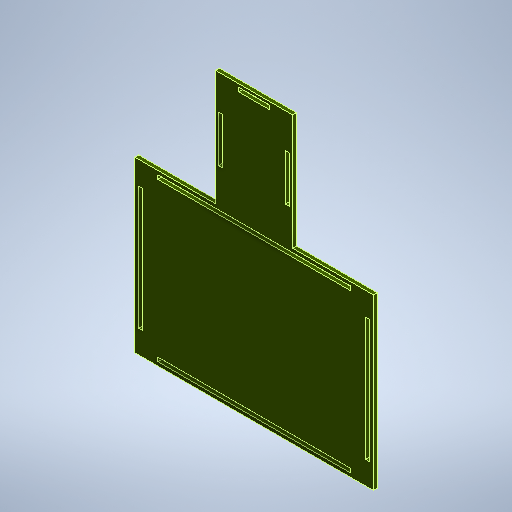
# Autodesk Inventor part: Finishing Sheets .5 ( Buttom )
Saved by Autodesk Inventor 2025.4 (Build 294407000, 407)
## iProperties
Created: 2026-04-04
Part Number: Finishing Sheets .5 ( Buttom )
Material: Generic
Document SubType Name: Sheet Metal
Designer: lenovo
Density: 1 g/cm^3
Sheet Metal Rule: Default_mm
Appearance: Default(1)
Author: lenovo
Autodesk Inventor part; units mm, degrees
ref_plane "YZ Plane" through (0, 0, 0) normal (1, 0, 0) x (0, 1, 0)
ref_plane "XZ Plane" through (0, 0, 0) normal (0, 1, 0) x (-1, 0, 0)
ref_plane "XY Plane" through (0, 0, 0) normal (0, 0, 1) x (1, 0, 0)
sketch "Sketch1" plane through (0, 0, 0) normal (0, 0, 1) x (1, 0, 0)
  line L0 (-155, -110) -> (155, -110)
  line L1 (155, -110) -> (155, 110)
  line L2 (155, 110) -> (-155, 110)
  line L3 (-155, 110) -> (-155, -110)
  line L4 (-155, -110) -> (155, 110) construction
  line L5 (155, -110) -> (-155, 110) construction
  line L6 (-125, 105) -> (125, 105)
  line L7 (125, 105) -> (125, 99.9)
  line L8 (125, 99.9) -> (-125, 99.9)
  line L9 (-125, 99.9) -> (-125, 105)
  line L10 (150, 80) -> (144.9, 80)
  line L11 (144.9, 80) -> (144.9, -80)
  line L12 (144.9, -80) -> (150, -80)
  line L13 (150, -80) -> (150, 80)
  line L14 (-155, 0) -> (155, 0)
  line L15 (0, 110) -> (0, -110)
  line L16 (-125, -105) -> (125, -105)
  line L17 (125, -105) -> (125, -99.9)
  line L18 (125, -99.9) -> (-125, -99.9)
  line L19 (-125, -99.9) -> (-125, -105)
  line L20 (-150, 80) -> (-144.9, 80)
  line L21 (-144.9, 80) -> (-144.9, -80)
  line L22 (-144.9, -80) -> (-150, -80)
  line L23 (-150, -80) -> (-150, 80)
  point P0 (0, 0)
  point P1 (0, 105)
  point P2 (144.9, 0)
  point P3 (0, -105)
  point P4 (-144.9, 0)
  dimension "d0" = 310
  dimension "d1" = 220
  dimension "d2" = 5.1
  dimension "d3" = 5.1
  dimension "d4" = 30
  dimension "d5" = 30
  dimension "d6" = 5
  dimension "d7" = 5
  measures "d0" distance of L2.end L1.end
  measures "d1" distance of L1.end L0.end
  measures "d2" distance between parallel lines of L6 L8
  measures "d3" distance of L10.start L10.end
  measures "d4" distance between parallel lines of L1 L7
  measures "d5" distance between parallel lines of L2 L10
  measures "d6" distance between parallel lines of L13 L1
  measures "d7" distance between parallel lines of L2 L6
extrude "Plate1" add sketch "Sketch1" along normal blind 5 contours L3 L14 L23 L22 L21 L15 L18 L19 L16 L0 | L15 L16 L17 L18 L14 L11 L12 L13 L1 L0 | L3 L2 L15 L6 L9 L8 L14 L21 L20 L23 | L14 L13 L10 L11 L15 L8 L7 L6 L2 L1
sketch "Sketch2" plane through (0, 0, 5) normal (0, 0, 1) x (1, 0, 0)
  line L0 (-50, 260) -> (50, 260)
  line L1 (50, 260) -> (50, 110)
  line L2 (50, 110) -> (-50, 110)
  line L3 (-50, 110) -> (-50, 260)
  line L4 (-155, 110) -> (155, 110)
  point P0 (0, 0)
  point P1 (0, 260)
  point P2 (0, 110)
  point P3 (0, 110)
  dimension "d9" = 100
  dimension "d10" = 150
  measures "d9" distance of L1.end L2.end
  measures "d10" distance of L0.end L1.end
sheet face with bend "Face2" sketch "Sketch2" thickness 5 toward (0, 0, -1) bend radius 5
bend "Bend1"
sketch "Sketch3" plane through (0, 0, 5) normal (0, 0, 1) x (1, 0, 0)
  line L0 (-20, 250.8) -> (20, 250.8)
  line L1 (20, 250.8) -> (20, 256)
  line L2 (20, 256) -> (-20, 256)
  line L3 (-20, 256) -> (-20, 250.8)
  line L4 (-20, 250.8) -> (20, 256) construction
  line L5 (20, 250.8) -> (-20, 256) construction
  line L6 (50, 260) -> (-50, 260) projected
  line L7 (-46, 155) -> (-40.8, 155)
  line L8 (-40.8, 155) -> (-40.8, 215)
  line L9 (-40.8, 215) -> (-46, 215)
  line L10 (-46, 215) -> (-46, 155)
  line L11 (-46, 155) -> (-40.8, 215) construction
  line L12 (-40.8, 155) -> (-46, 215) construction
  line L13 (-50, 260) -> (-50, 110) projected
  line L14 (-125, 105) -> (125, 105) projected
  line L15 (0, 105) -> (0, 260)
  line L16 (46, 155) -> (40.8, 155)
  line L17 (40.8, 155) -> (40.8, 215)
  line L18 (40.8, 215) -> (46, 215)
  line L19 (46, 215) -> (46, 155)
  line L20 (46, 155) -> (40.8, 215) construction
  line L21 (40.8, 155) -> (46, 215) construction
  point P0 (0, 0)
  point P1 (0, 253.4)
  point P2 (-43.4, 185)
  point P3 (-50, 185)
  point P4 (43.4, 185)
  dimension "d16" = 5.2
  dimension "d17" = 4
  dimension "d18" = 40
  dimension "d19" = 5.2
  dimension "d20" = 60
  dimension "d21" = 4
  constraints: 38 end point, 7 midpoint, 5 symmetric about line, 4 parallel, 3 perpendicular, 2 horizontal, 1 horizontal alignment, 1 vertical alignment
  measures "d16" distance of L0.end L1.end
  measures "d17" distance between parallel lines of L2 L6
  measures "d18" distance of L1.end L2.end
  measures "d19" distance of L8.end L9.end
  measures "d20" distance of L7.end L8.end
  measures "d21" distance between parallel lines of L13 L10
extrude "Cut1" cut sketch "Sketch3" against normal blind 5
feature "Corner Round1" [suppressed]
equation "\"d7\" = d6"
equation "\"d21\" = d17"
equation "\"d22\" = Thickness"
equation "\"d8\" = Thickness"
equation "\"d11\" = BendRadius"
equation "\"d12\" = BendReliefWidth"
equation "\"d14\" = MinimumRemnant"
equation "\"d13\" = BendReliefDepth"
equation "\"d15\" = TransitionRadius"
equation "\"BendRadius\" = Thickness"
equation "\"BendReliefWidth\" = Thickness"
equation "\"BendReliefDepth\" = 0.5 * Thickness"
equation "\"TransitionRadius\" = BendRadius"
equation "\"JacobiRadiusSize\" = BendRadius"
equation "\"GapSize\" = Thickness"
equation "\"Thickness\" = 5"
equation "\"MinimumRemnant\" = 10"
body "Solid1"
